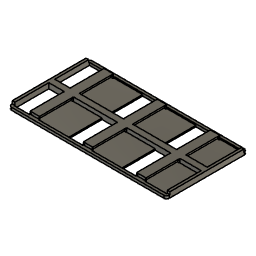
Center Cover 2x3 v8 (Autodesk Fusion 360 design; units mm, degrees)
Autodesk Fusion 360 part; units mm, degrees
sketch "Schizzo1" plane through (0, 0, 0) normal (0, 0, 1) x (1, 0, 0)
  line L0 (50, 150) -> (168.7, 150) construction
  line L1 (168.7, 150) -> (168.7, 89.3) construction
  line L2 (168.7, 89.3) -> (50, 89.3) construction
  line L3 (50, 89.3) -> (50, 150) construction
  line L4 (50, 119.65) -> (168.7, 119.65) construction
  line L5 (109.35, 150) -> (109.35, 89.3) construction
  line L6 (168.6, 89.4) -> (50.1, 89.4)
  line L7 (50.1, 89.4) -> (50.1, 149.9)
  line L8 (50.1, 149.9) -> (168.6, 149.9)
  line L9 (168.6, 149.9) -> (168.6, 89.4)
  line L10 (168.6, 89.4) -> (50.1, 149.9) construction
  line L11 (50.1, 89.4) -> (168.6, 149.9) construction
  point P0 (109.35, 119.65)
  dimension "d1" = 118.7
  dimension "d2" = 60.7
  dimension "d3" = 0.1
  dimension "d4" = 0.1
  constraint horizontal L0
  constraint vertical L1
  constraint horizontal L2
  constraint vertical L3
  constraint midpoint L3 L4.start
  constraint midpoint L1 L4.end
  constraint midpoint L0 L5.start
  constraint midpoint L2 L5.end
  constraint horizontal L6
  constraint perpendicular L6 L7
  constraint parallel L6 L8
  constraint parallel L7 L9
  constraint coincident L10 P0
  constraint coincident L11 P0
  constraint midpoint L4 P0
  measures "d1" distance of L0.start L0.end
  measures "d2" distance of L0 L2
  measures "d3" distance of L3 L7
  measures "d4" distance of L0 L8
extrude "Estrusione1" add sketch "Schizzo1" along normal blind 4
fillet "Raccordo1" radius 2 4 edges at (50.1, 89.4, 2) (168.6, 89.4, 2) (50.1, 149.9, 2) (168.6, 149.9, 2)
sketch "Schizzo2" plane through (0, 0, 4) normal (0, 0, 1) x (-1, 0, 0)
  arc A0 (-168.6, -147.9) -> (-166.6, -149.9) centre (-166.6, -147.9) ccw
  line L0 (-166.6, -149.9) -> (-52.1, -149.9)
  arc A1 (-52.1, -149.9) -> (-50.1, -147.9) centre (-52.1, -147.9) ccw
  line L1 (-50.1, -147.9) -> (-50.1, -91.4)
  arc A2 (-50.1, -91.4) -> (-52.1, -89.4) centre (-52.1, -91.4) ccw
  line L2 (-52.1, -89.4) -> (-166.6, -89.4)
  arc A3 (-166.6, -89.4) -> (-168.6, -91.4) centre (-166.6, -91.4) ccw
  line L3 (-168.6, -91.4) -> (-168.6, -147.9)
  line L4 (-50.1, -149.9) -> (-168.6, -149.9) construction
  line L5 (-168.6, -149.9) -> (-168.6, -89.4) construction
  line L6 (-168.6, -89.4) -> (-50.1, -89.4) construction
  line L7 (-50.1, -89.4) -> (-50.1, -149.9) construction
  line L8 (-50.1, -119.65) -> (-168.6, -119.65) construction
  line L9 (-109.35, -149.9) -> (-109.35, -89.4) construction
  line L10 (-166.6, -91.4) -> (-52.1, -91.4)
  line L11 (-52.1, -91.4) -> (-52.1, -147.9)
  line L12 (-52.1, -147.9) -> (-166.6, -147.9)
  line L13 (-166.6, -147.9) -> (-166.6, -91.4)
  line L14 (-166.6, -91.4) -> (-52.1, -147.9) construction
  line L15 (-52.1, -91.4) -> (-166.6, -147.9) construction
  line L16 (-70.6, -91.4) -> (-70.6, -147.9)
  line L17 (-63.6, -147.9) -> (-63.6, -91.4)
  line L18 (-52.1, -147.9) -> (-62.1, -147.9)
  line L19 (-62.1, -147.9) -> (-62.1, -121.9)
  line L20 (-62.1, -121.9) -> (-52.1, -121.9)
  line L21 (-52.1, -121.9) -> (-52.1, -147.9)
  line L22 (-102.1, -147.9) -> (-102.1, -121.9)
  line L23 (-102.1, -121.9) -> (-92.1, -121.9)
  line L24 (-92.1, -121.9) -> (-92.1, -147.9)
  line L25 (-92.1, -147.9) -> (-102.1, -147.9)
  line L26 (-142.1, -147.9) -> (-142.1, -121.9)
  line L27 (-142.1, -121.9) -> (-132.1, -121.9)
  line L28 (-132.1, -121.9) -> (-132.1, -147.9)
  line L29 (-132.1, -147.9) -> (-142.1, -147.9)
  line L30 (-62.1, -117.4) -> (-62.1, -91.4)
  line L31 (-62.1, -91.4) -> (-52.1, -91.4)
  line L32 (-52.1, -91.4) -> (-52.1, -117.4)
  line L33 (-52.1, -117.4) -> (-62.1, -117.4)
  line L34 (-102.1, -117.4) -> (-102.1, -91.4)
  line L35 (-102.1, -91.4) -> (-92.1, -91.4)
  line L36 (-92.1, -91.4) -> (-92.1, -117.4)
  line L37 (-92.1, -117.4) -> (-102.1, -117.4)
  line L38 (-142.1, -117.4) -> (-142.1, -91.4)
  line L39 (-142.1, -91.4) -> (-132.1, -91.4)
  line L40 (-132.1, -91.4) -> (-132.1, -117.4)
  line L41 (-132.1, -117.4) -> (-142.1, -117.4)
  line L42 (-103.6, -147.9) -> (-103.6, -91.4)
  line L43 (-110.6, -147.9) -> (-110.6, -91.4)
  line L44 (-143.6, -147.9) -> (-143.6, -91.4)
  line L45 (-150.6, -147.9) -> (-150.6, -91.4)
  line L46 (-52.1, -121.9) -> (-166.6, -121.9)
  line L47 (-52.1, -117.4) -> (-166.6, -117.4)
  point P0 (-109.35, -119.65)
  point P1 (-109.35, -119.65)
  dimension "d9" = 2
  dimension "d10" = 2
  dimension "d11" = 7
  dimension "d14" = 10
  dimension "d15" = 26
  dimension "d18" = -40
  dimension "d19" = 30.5
  dimension "d20" = 7
  dimension "d21" = 1.5
  dimension "d22" = 1.5
  dimension "d25" = 7
  dimension "d26" = 1.5
  constraint horizontal L4
  constraint vertical L5
  constraint horizontal L6
  constraint vertical L7
  constraint collinear L0 L4
  constraint collinear L1 L7
  constraint collinear L2 L6
  constraint collinear L3 L5
  constraint midpoint L7 L8.start
  constraint midpoint L5 L8.end
  constraint midpoint L4 L9.start
  constraint midpoint L6 L9.end
  constraint horizontal L10
  constraint perpendicular L10 L11
  constraint parallel L10 L12
  constraint parallel L11 L13
  constraint coincident L14 P1
  constraint coincident L15 P1
  constraint midpoint L9 P1
  constraint parallel L16 L17
  constraint coincident P1 P0
  constraint horizontal L18
  constraint vertical L19
  constraint horizontal L20
  constraint vertical L21
  constraint coincident A1.centre L11.end
  constraint coincident L12 L42.start
  constraint coincident L10 L42.end
  constraint perpendicular L10 L42
  constraint coincident L12 L43.start
  constraint coincident L10 L43.end
  constraint perpendicular L10 L43
  constraint coincident L12 L44.start
  constraint coincident L10 L44.end
  constraint perpendicular L10 L44
  constraint coincident L12 L45.start
  constraint coincident L10 L45.end
  constraint perpendicular L10 L45
  constraint coincident L13 L46.end
  constraint perpendicular L13 L46
  constraint symmetric L8 L20.end L32.end
  constraint symmetric L8 L46.end L47.end
  measures "d9" distance of L4 L12
  measures "d10" distance of L7 L11
  measures "d11" distance of L16.end L17.start
  measures "d14" distance of A1.centre L18.end
  measures "d15" distance of A1.centre L20.end
  measures "d20" distance of L42 L43
  measures "d21" distance of L17 L19
  measures "d22" distance of L22 L42
  measures "d25" distance of L44 L45
  measures "d26" distance of L26 L44
extrude "Estrusione2" cut sketch "Schizzo2" against normal blind 3 contours L10 L13 L45 L47 | L10 L38 L44 L47 | L12 L13 L45 L46 | L10 L38 L39 L40 L41 L47 | L10 L40 L43 L47 | L12 L26 L44 L46 | L12 L26 L27 L28 L29 L46 | L10 L34 L42 L47 | L12 L28 L43 L46 | L10 L34 L35 L36 L37 L47 | L10 L16 L36 L47 | L12 L22 L42 L46 | L12 L22 L23 L24 L25 L46 | L10 L17 L30 L47 | L12 L16 L24 L46 | L10 L11 L30 L31 L32 L33 L47 | L12 L17 L19 L46 | L11 L12 L18 L19 L20 L21 L46
extrude "Estrusione3" cut sketch "Schizzo2" against normal blind 4 contours L10 L38 L39 L40 L41 L47 | L12 L26 L27 L28 L29 L46 | L10 L34 L35 L36 L37 L47 | L12 L22 L23 L24 L25 L46 | L10 L11 L30 L31 L32 L33 L47 | L11 L12 L18 L19 L20 L21 L46
ref_plane "Piano di lavoro1" through (109.35, 119.65, 4) normal (0, -1, 0) x (1, 0, 0)
sketch "Schizzo3" plane through (0, 119.65, 0) normal (0, -1, 0) x (-1, 0, 0)
  line L0 (-50.1, -4) -> (-168.7, -4) construction
  line L1 (-168.7, -4) -> (-168.7, 0) construction
  line L2 (-168.7, 0) -> (-50.1, 0) construction
  line L3 (-50.1, 0) -> (-50.1, -4) construction
  line L4 (-168.6, -4) -> (-50.1, -4) construction
  line L5 (-50.1, -1) -> (-168.7, -1) construction
  line L6 (-110.6, -1) -> (-132.1, -1) construction
  line L7 (-63.6, -4) -> (-63.6, 0) construction
  line L8 (-70.6, -4) -> (-70.6, 0) construction
  line L9 (-63.6, -4) -> (-63.6, -1) construction
  line L10 (-70.6, -4) -> (-70.6, -1) construction
  line L11 (-103.6, -4) -> (-103.6, 0) construction
  line L12 (-110.6, -4) -> (-110.6, 0) construction
  line L13 (-103.6, -4) -> (-103.6, -1) construction
  line L14 (-110.6, -4) -> (-110.6, -1) construction
  line L15 (-143.6, -4) -> (-143.6, 0) construction
  line L16 (-150.6, -4) -> (-150.6, 0) construction
  line L17 (-143.6, -4) -> (-143.6, -1) construction
  line L18 (-150.6, -4) -> (-150.6, -1) construction
  line L19 (-63.6, -4) -> (-65.3321, -1)
  line L20 (-63.6, -4) -> (-60.1359, -4) construction
  line L21 (-70.6, -4) -> (-68.8679, -1)
  line L22 (-70.6, -4) -> (-67.1359, -4) construction
  line L23 (-63.6, -4) -> (-63.6, -1)
  line L24 (-63.6, -1) -> (-65.3321, -1)
  line L25 (-68.8679, -1) -> (-70.6, -1)
  line L26 (-70.6, -1) -> (-70.6, -4)
  line L27 (-103.6, -1) -> (-103.6, -4)
  line L28 (-103.6, -4) -> (-105.3321, -1)
  line L29 (-105.3321, -1) -> (-103.6, -1)
  line L30 (-110.6, -1) -> (-110.6, -4)
  line L31 (-110.6, -4) -> (-108.8679, -1)
  line L32 (-108.8679, -1) -> (-110.6, -1)
  line L33 (-143.6, -1) -> (-143.6, -4)
  line L34 (-143.6, -4) -> (-145.3321, -1)
  line L35 (-145.3321, -1) -> (-143.6, -1)
  line L36 (-150.6, -1) -> (-150.6, -4)
  line L37 (-150.6, -4) -> (-148.8679, -1)
  line L38 (-148.8679, -1) -> (-150.6, -1)
  point P0 (-168.7, 0)
  dimension "d28" = 120
  dimension "d29" = 60
  dimension "d30" = 30
  dimension "d31" = 30
  dimension "d32" = 30
  dimension "d33" = 30
  constraint horizontal L0
  constraint vertical L1
  constraint horizontal L2
  constraint vertical L3
  constraint coincident L0.start L3.end
  constraint coincident P0 L1.end
  constraint coincident L3 L5.start
  constraint coincident L1 L5.end
  constraint perpendicular L1 L5
  constraint collinear L5 L6
  constraint coincident L4 L7.start
  constraint coincident L2 L7.end
  constraint perpendicular L2 L7
  constraint coincident L0 L8.start
  constraint coincident L2 L8.end
  constraint perpendicular L2 L8
  constraint collinear L7 L9
  constraint collinear L8 L10
  constraint coincident L0 L11.start
  constraint coincident L2 L11.end
  constraint perpendicular L2 L11
  constraint coincident L0 L12.start
  constraint coincident L2 L12.end
  constraint perpendicular L2 L12
  constraint collinear L11 L13
  constraint collinear L12 L14
  constraint coincident L0 L15.start
  constraint coincident L2 L15.end
  constraint perpendicular L2 L15
  constraint coincident L0 L16.start
  constraint coincident L2 L16.end
  constraint perpendicular L2 L16
  constraint collinear L15 L17
  constraint collinear L16 L18
  constraint horizontal L20
  constraint coincident L5 L19.end
  constraint horizontal L22
  constraint coincident L8.start L10.start
  constraint coincident L5 L21.end
  constraint coincident L9.end L23.end
  constraint coincident L10.end L25.end
  constraint coincident L13.end L27.start
  constraint coincident L11.start L13.start
  constraint coincident L5 L28.end
  constraint coincident L6.start L14.end
  constraint coincident L12.start L14.start
  constraint coincident L5 L31.end
  constraint coincident L17.end L33.start
  constraint coincident L15.start L17.start
  constraint coincident L5 L34.end
  constraint coincident L18.end L36.start
  constraint coincident L16.start L18.start
  constraint coincident L5 L37.end
  measures "d28" angle of L19 L20
  measures "d29" angle of L21 L22
  measures "d30" angle of L27 L28
  measures "d31" angle of L30 L31
  measures "d32" angle of L33 L34
  measures "d33" angle of L36 L37
extrude "Estrusione4" cut sketch "Schizzo3" along normal blind 25 from surface at 2.5
extrude "Estrusione6" cut sketch "Schizzo3" against normal blind 25 from surface at -2.5
sketch "Schizzo4" plane through (0, 0, 4) normal (0, 0, 1) x (-1, 0, 0)
  line L0 (-50.1, -149.9) -> (-168.6, -149.9) construction
  line L1 (-168.6, -149.9) -> (-168.6, -89.4) construction
  line L2 (-168.6, -89.4) -> (-50.1, -89.4) construction
  line L3 (-50.1, -89.4) -> (-50.1, -149.9) construction
  line L4 (-166.6, -149.9) -> (-52.1, -149.9) construction
  line L5 (-168.6, -91.4) -> (-168.6, -147.9) construction
  line L6 (-50.1, -147.9) -> (-50.1, -91.4) construction
  line L7 (-52.1, -89.4) -> (-166.6, -89.4) construction
  line L8 (-50.1, -149.9) -> (-168.6, -149.9)
  line L9 (-168.6, -149.9) -> (-168.6, -147.4)
  line L10 (-168.6, -147.4) -> (-50.1, -147.4)
  line L11 (-50.1, -147.4) -> (-50.1, -149.9)
  line L12 (-50.1, -119.65) -> (-168.6, -119.65) construction
  line L13 (-50.1, -91.9) -> (-168.6, -91.9)
  line L14 (-168.6, -91.9) -> (-168.6, -89.4)
  line L15 (-168.6, -89.4) -> (-50.1, -89.4)
  line L16 (-50.1, -89.4) -> (-50.1, -91.9)
  dimension "d36" = 2.5
  dimension "d37" = 2.5
  constraint horizontal L0
  constraint vertical L1
  constraint horizontal L2
  constraint vertical L3
  constraint collinear L0 L4
  constraint collinear L1 L5
  constraint collinear L3 L6
  constraint collinear L2 L7
  constraint horizontal L8
  constraint vertical L9
  constraint horizontal L10
  constraint vertical L11
  constraint coincident L5 L9.end
  constraint midpoint L3 L12.start
  constraint midpoint L5 L12.end
  constraint horizontal L13
  constraint vertical L14
  constraint horizontal L15
  constraint vertical L16
  constraint coincident L3 L13.start
  measures "d36" distance of L0.start L10.end
  measures "d37" distance of L13 L15
extrude "Estrusione5" cut sketch "Schizzo4" against normal blind 2
equation "d28 = 90 deg + 30 deg"
equation "d37 = d36"
